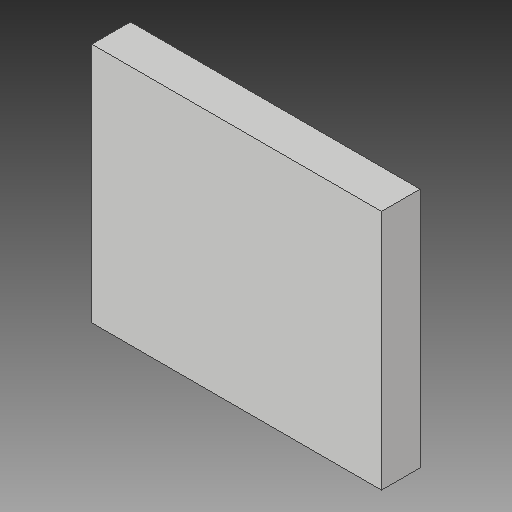
# Autodesk Inventor part: USBブリッジ基板2
Saved by Autodesk Inventor 2017 (Build 210142000, 142)
## iProperties
Created: 2016-08-22
Part Number: USBブリッジ基板2
Material: 一般
Document SubType Name: Modeling
Designer: NN
Density: 1 g/cm^3
Appearance: 既定
Mass: 0.192 g
Surface Area: 3.104 cm^2
Volume: 0.192 cm^3
Author: NN
Autodesk Inventor part; units mm, degrees
ref_plane "YZ Plane" through (0, 0, 0) normal (1, 0, 0) x (0, 1, 0)
ref_plane "XZ Plane" through (0, 0, 0) normal (0, 1, 0) x (-1, 0, 0)
ref_plane "XY Plane" through (0, 0, 0) normal (0, 0, 1) x (1, 0, 0)
sketch "スケッチ1" plane through (0, 0, 0) normal (0, 0, 1) x (1, 0, 0)
  line L0 (0, 0) -> (12, 0)
  line L1 (12, 0) -> (12, 10)
  line L2 (12, 10) -> (0, 10)
  line L3 (0, 10) -> (0, 0)
  dimension "d0" = 12
  dimension "d1" = 10
  constraints: 8 end point, 2 parallel, 1 horizontal, 1 perpendicular
  measures "d0" distance of L0.start L0.end
  measures "d1" distance of L2.end L0.start
extrude "押し出し1" add sketch "スケッチ1" along normal blind 1.6
